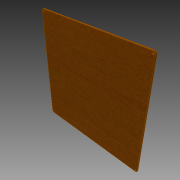
# Autodesk Inventor part: heatbed_thermal_insulation
Saved by Autodesk Inventor 2014 (Build 180170000, 170)
## iProperties
Created: 2014-03-29
Part Number: heatbed_thermal_insulation
Material: Wood
Document SubType Name: Modeling
Designer: buben
Density: 0.570257 g/cm^3
Appearance: Yellow Pine - Solid Natural Low Gloss
Author: buben
Autodesk Inventor part; units mm, degrees
ref_plane "YZ Plane" through (0, 0, 0) normal (1, 0, 0) x (0, 1, 0)
ref_plane "XZ Plane" through (0, 0, 0) normal (0, 1, 0) x (-1, 0, 0)
ref_plane "XY Plane" through (0, 0, 0) normal (0, 0, 1) x (1, 0, 0)
sketch "Sketch1" plane through (0, 0, 0) normal (0, 1, 0) x (-1, 0, 0)
  line L0 (-2, 0) -> (-214, 0)
  line L1 (-216, -2) -> (-216, -214)
  line L2 (-214, -216) -> (-2, -216)
  line L3 (0, -214) -> (0, -2)
  line L4 (0, -214) -> (-2, -216)
  line L5 (-216, -214) -> (-214, -216)
  line L6 (-216, -2) -> (-214, 0)
  line L7 (-2, 0) -> (0, -2)
  line L8 (-3.5, -212.5) -> (-212.5, -212.5) construction
  line L9 (-212.5, -212.5) -> (-212.5, -3.5) construction
  line L10 (-212.5, -3.5) -> (-3.5, -3.5) construction
  line L11 (-3.5, -3.5) -> (-3.5, -212.5) construction
  circle A0 centre (-3.5, -3.5) radius 1.6
  circle A1 centre (-3.5, -212.5) radius 1.6
  circle A2 centre (-212.5, -212.5) radius 1.6
  circle A3 centre (-212.5, -3.5) radius 1.6
  point P0 (0, 0)
  point P1 (-216, -216)
  point P2 (-216, 0)
  point P3 (0, -216)
  point P4 (-108, -212.5)
  point P5 (-108, -216)
  point P6 (-212.5, -108)
  point P7 (-216, -108)
  dimension "d0" = 2
  dimension "d1" = 2
  dimension "d2" = 2
  dimension "d3" = 2
  dimension "d4" = 2
  dimension "d5" = 2
  dimension "d6" = 2
  dimension "d7" = 2
  dimension "d8" = 216
  dimension "d9" = 209
  dimension "d10" = 3.2
  constraints: 24 end point, 8 point on line, 4 centre point, 4 coincident, 4 midpoint, 4 parallel, 4 perpendicular, 3 equal radius, 2 horizontal, 1 horizontal alignment, 1 vertical alignment
  measures "d0" distance of L3.start point (0, -216)
  measures "d1" distance of L2.end point (0, -216)
  measures "d2" distance of L1.end point (-216, -216)
  measures "d3" distance of L2.start point (-216, -216)
  measures "d4" distance of L1.start point (-216, 0)
  measures "d5" distance of L0.end point (-216, 0)
  measures "d6" distance of L0.start point (0, 0)
  measures "d7" distance of L3.end point (0, 0)
  measures "d8" distance between parallel lines of L1 L3
  measures "d9" distance of L9.end L10.end
  measures "d10" diameter of A1
extrude "Extrusion1" add sketch "Sketch1" along normal blind 3
equation "\"d1\" = d0"
equation "\"d2\" = d0"
equation "\"d3\" = d2"
equation "\"d4\" = d0"
equation "\"d5\" = d4"
equation "\"d6\" = d0"
equation "\"d7\" = d6"
body "Solid1"
